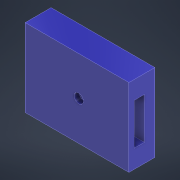
# Autodesk Inventor part: Каменъ
Saved by Autodesk Inventor 2021.2 (Build 252289000, 289)
## iProperties
Created: 2021-05-30
Part Number: Каменъ
Material: Типовые
Document SubType Name: Modeling
Designer: Admin
Density: 1 g/cm^3
Appearance: Гладкий — темно-синий
Mass: 1172.37 g
Surface Area: 1324.79 cm^2
Volume: 1172.37 cm^3
Author: Admin
Autodesk Inventor part; units mm, degrees
ref_plane "YZ Plane" through (0, 0, 0) normal (1, 0, 0) x (0, 1, 0)
ref_plane "XZ Plane" through (0, 0, 0) normal (0, 1, 0) x (-1, 0, 0)
ref_plane "XY Plane" through (0, 0, 0) normal (0, 0, 1) x (1, 0, 0)
sketch "Эскиз1" plane through (0, 0, 0) normal (0, 0, 1) x (1, 0, 0)
  line L0 (0, 0) -> (200, 0)
  line L1 (200, 0) -> (200, 150)
  line L2 (200, 150) -> (0, 150)
  line L3 (0, 150) -> (0, 0)
  dimension "d0" = 200
  dimension "d1" = 150
  constraints: 8 end point, 2 parallel, 1 horizontal, 1 perpendicular
  measures "d0" distance of L2.end L1.end
  measures "d1" distance of L1.end L0.end
extrude "Выдавливание1" add sketch "Эскиз1" along normal blind 50
sketch "Эскиз2" plane through (200, 0, 0) normal (1, 0, 0) x (0, 0, -1)
  line L0 (-40, 115.1107) -> (-20, 115.1107)
  line L1 (-20, 115.1107) -> (-20, 35.1107)
  line L2 (-20, 35.1107) -> (-40, 35.1107)
  line L3 (-40, 35.1107) -> (-40, 115.1107)
  line L4 (0, 0) -> (0, 150) projected
  line L5 (-50, 0) -> (-50, 150) projected
  line L6 (-20, 35.1107) -> (-21.2634, 0)
  line L7 (0, 0) -> (-50, 0) projected
  line L8 (-20, 115.1107) -> (-15.8659, 150)
  line L9 (0, 150) -> (-50, 150) projected
  dimension "d4" = 20
  dimension "d5" = 80
  dimension "d15" = 20
  constraints: 12 end point, 3 point on line, 2 parallel, 1 equal length, 1 horizontal, 1 perpendicular
  measures "d4" distance of L0.start L0.end
  measures "d5" distance of L0.end L1.end
  measures "d15" distance between parallel lines of L4 L1
extrude "Выдавливание2" cut sketch "Эскиз2" against normal through all contours L0 L1 L2 L3
sketch "Эскиз3" plane through (0, 0, 0) normal (0, 0, -1) x (-1, 0, 0)
  line L0 (-200, 150) -> (0, 150) projected
  line L1 (-103.2089, 150) -> (-103.2089, 75)
  line L2 (0, 0) -> (-200, 0) projected
  line L3 (-103.2089, 75) -> (-6.4177, 75)
  line L4 (-103.2089, 75) -> (-200, 75)
  line L5 (-200, 115.1107) -> (-200, 35.1107) projected
  line L6 (-103.2089, 75) -> (-103.2089, 0)
  line L7 (-200, 0) -> (-200, 150) projected
  line L8 (0, 0) -> (-200, 0) projected
  constraints: 8 end point, 2 collinear, 2 horizontal, 2 point on line, 2 vertical, 1 midpoint
hole "Отверстие1" at (103.2089, 75, 0) direction (0, 0, 1) diameter 18 end through all
